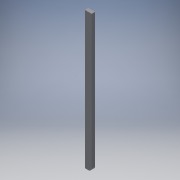
# Autodesk Inventor part: Plexi hook
Saved by Autodesk Inventor 2019 (Build 230136000, 136)
## iProperties
Created: 2019-02-17
Part Number: Plexi hook
Material: Generic
Document SubType Name: Modeling
Designer: josh
Density: 1 g/cm^3
Appearance: Default
Author: josh
Autodesk Inventor part; units mm, degrees
ref_plane "YZ Plane" through (0, 0, 0) normal (1, 0, 0) x (0, 1, 0)
ref_plane "XZ Plane" through (0, 0, 0) normal (0, 1, 0) x (-1, 0, 0)
ref_plane "XY Plane" through (0, 0, 0) normal (0, 0, 1) x (1, 0, 0)
sketch "Sketch1" plane through (0, 0, 0) normal (0, 0, 1) x (1, 0, 0)
  line L0 (0, 0) -> (3.175, 0)
  line L1 (6.35, 3.175) -> (6.35, 127)
  line L2 (6.35, 127) -> (0, 127)
  line L3 (0, 127) -> (0, 0)
  arc A0 (3.175, 0) -> (6.35, 3.175) centre (3.175, 3.175) ccw
  line L4 (0, 0) -> (-101.6, 0)
  line L5 (-101.6, 0) -> (-101.6, 3.175)
  point P0 (6.35, 0)
  dimension "d0" = 6.35
  dimension "d1" = 127
  dimension "d2" = 3.175
  dimension "d5" = 101.6
  dimension "d6" = 3.175
  constraints: 12 end point, 2 horizontal, 2 parallel, 2 point on circle, 2 point on line, 2 tangent, 1 centre point, 1 perpendicular, 1 vertical
  measures "d0" distance of L2.end L1.end
  measures "d1" distance of L1.end point (6.35, 0)
  measures "d2" radius of A0
  measures "d5" distance of L0.start L4.end
  measures "d6" distance of L4.end L5.end
extrude "Extrusion1" add sketch "Sketch1" along normal blind 3.175
body "Solid1"
